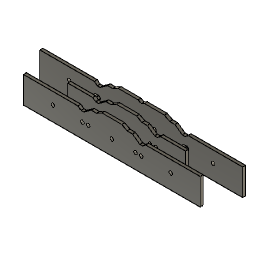
Spur_0_Module_Kopfstuecke_v3 (Autodesk Fusion 360 design; units mm, degrees)
Autodesk Fusion 360 part; units mm, degrees
sketch "Skizze1" plane through (0, 0, 0) normal (0, 1, 0) x (1, 0, 0) in component "FREMO_600mm"
  line L0 (0, 0) -> (0, -110) construction
  line L1 (0, 0) -> (-300, 0)
  line L2 (-300, 0) -> (-300, -90)
  line L3 (-300, -90) -> (-115, -90)
  line L4 (0, -110) -> (-34, -110)
  line L5 (-34, -110) -> (-52, -100)
  line L6 (-52, -100) -> (-70, -100)
  line L7 (-70, -100) -> (-95, -82)
  line L8 (-95, -82) -> (-105, -82)
  line L9 (-105, -82) -> (-115, -90)
  line L10 (-300, -50) -> (0, -50) construction
  circle A0 centre (-100, -50) radius 6
  circle A1 centre (-80, -50) radius 6
  circle A2 centre (-200, -50) radius 6
  line L11 (0, -110) -> (34, -110)
  line L12 (34, -110) -> (52, -100)
  line L13 (52, -100) -> (70, -100)
  line L14 (70, -100) -> (95, -82)
  line L15 (95, -82) -> (105, -82)
  line L16 (105, -82) -> (115, -90)
  line L17 (300, -90) -> (115, -90)
  line L18 (300, 0) -> (300, -90)
  line L19 (0, 0) -> (300, 0)
  circle A3 centre (200, -50) radius 6
  circle A4 centre (100, -50) radius 6
  circle A5 centre (80, -50) radius 6
  circle A6 centre (0, -50) radius 6
  dimension "d13" = 34
  dimension "d14" = 18
  dimension "d15" = 18
  dimension "d16" = 10
  dimension "d17" = 25
  dimension "d18" = 10
  dimension "d19" = 10
  dimension "d20" = 100
  dimension "d21" = 90
  dimension "d22" = 8
  dimension "d23" = 300
  dimension "d24" = 12
  dimension "d25" = 12
  dimension "d26" = 12
  dimension "d27" = 50
  dimension "d28" = 80
  dimension "d29" = 100
  dimension "d30" = 200
  dimension "d31" = 12
  constraint coincident L0.start L1.start
  constraint vertical L0
  constraint perpendicular L0 L1
  constraint perpendicular L1 L2
  constraint perpendicular L0 L4
  constraint parallel L4 L6
  constraint parallel L6 L8
  constraint parallel L3 L8
  constraint coincident L2 L10.start
  constraint coincident L0 L10.end
  constraint perpendicular L0 L10
  constraint coincident L10 A0.centre
  constraint coincident L10 A1.centre
  constraint coincident L10 A2.centre
  constraint symmetric L4.start L0 L11.start
  constraint symmetric L0 L1.start L19.start
  constraint symmetric L0 L1.end L18.start
  constraint symmetric L0 L2.end L17.start
  constraint symmetric L0 L3.end L16.end
  constraint symmetric L0 L4.end L11.end
  constraint symmetric L0 L5.end L12.end
  constraint symmetric L0 L6.end L13.end
  constraint symmetric L0 L7.end L14.end
  constraint symmetric L0 L8.end L15.end
  constraint symmetric L0 A0 A4
  constraint symmetric L0 A1 A5
  constraint symmetric L0 A2 A3
  constraint coincident L10.end A6.centre
  measures "d13" distance of L0.end L4.end
  measures "d14" horizontal distance of L4.end L5.end
  measures "d15" distance of L5.end L6.end
  measures "d16" distance of L4 L6
  measures "d17" horizontal distance of L6.end L7.end
  measures "d18" distance of L7.end L8.end
  measures "d19" horizontal distance of L3.end L8.end
  measures "d20" distance of L1 L6
  measures "d21" distance of L1 L3
  measures "d22" distance of L3 L8
  measures "d23" distance of L0 L2
  measures "d24" diameter of A0
  measures "d25" diameter of A1
  measures "d26" diameter of A2
  measures "d27" distance of L1 L10
  measures "d28" distance of L0 A1.centre
  measures "d29" distance of L0 A0.centre
  measures "d30" distance of L0 A2.centre
  measures "d31" diameter of A6
extrude "Extrusion1" add sketch "Skizze1" along normal blind 10 makes body 1 in component "FREMO_600mm"
sketch "Skizze2" plane through (0, 0, 0) normal (0, 1, 0) x (1, 0, 0) in component "FREMO_400mm"
  line L0 (0, 0) -> (0, -110) construction
  line L1 (0, 0) -> (-200, 0)
  line L2 (-200, 0) -> (-200, -90)
  line L3 (-200, -90) -> (-115, -90)
  line L4 (-115, -90) -> (-105, -82)
  line L5 (-105, -82) -> (-95, -82)
  line L6 (-95, -82) -> (-70, -100)
  line L7 (-70, -100) -> (-52, -100)
  line L8 (-52, -100) -> (-34, -110)
  line L9 (-34, -110) -> (0, -110)
  line L10 (-200, -50) -> (0, -50) construction
  circle A0 centre (-100, -50) radius 6
  circle A1 centre (-80, -50) radius 6
  line L11 (34, -110) -> (0, -110)
  line L12 (52, -100) -> (34, -110)
  line L13 (70, -100) -> (52, -100)
  line L14 (95, -82) -> (70, -100)
  line L15 (105, -82) -> (95, -82)
  line L16 (115, -90) -> (105, -82)
  line L17 (200, -90) -> (115, -90)
  line L18 (200, 0) -> (200, -90)
  line L19 (0, 0) -> (200, 0)
  circle A2 centre (100, -50) radius 6
  circle A3 centre (80, -50) radius 6
  circle A4 centre (0, -50) radius 6
  dimension "d52" = 34
  dimension "d53" = 18
  dimension "d54" = 18
  dimension "d55" = 25
  dimension "d56" = 10
  dimension "d57" = 10
  dimension "d58" = 10
  dimension "d59" = 100
  dimension "d60" = 90
  dimension "d61" = 8
  dimension "d62" = 200
  dimension "d63" = 50
  dimension "d64" = 12
  dimension "d65" = 12
  dimension "d66" = 80
  dimension "d67" = 100
  dimension "d68" = 12
  constraint coincident L0.start L1.start
  constraint vertical L0
  constraint perpendicular L0 L1
  constraint perpendicular L1 L2
  constraint perpendicular L0 L9
  constraint parallel L7 L9
  constraint parallel L5 L7
  constraint parallel L3 L5
  constraint coincident L2 L10.start
  constraint coincident L0 L10.end
  constraint perpendicular L0 L10
  constraint coincident L10 A0.centre
  constraint coincident L10 A1.centre
  constraint symmetric L9.end L0 L11.end
  constraint symmetric L0 L1.start L19.start
  constraint symmetric L0 L1.end L18.start
  constraint symmetric L0 L2.end L17.start
  constraint symmetric L0 L3.end L16.start
  constraint symmetric L0 L4.end L15.start
  constraint symmetric L0 L5.end L14.start
  constraint symmetric L0 L6.end L13.start
  constraint symmetric L0 L7.end L12.start
  constraint symmetric L0 L8.end L11.start
  constraint symmetric L0 A0 A2
  constraint symmetric L0 A1 A3
  constraint coincident L10.end A4.centre
  measures "d52" distance of L0.end L8.end
  measures "d53" horizontal distance of L7.end L8.end
  measures "d54" distance of L6.end L7.end
  measures "d55" horizontal distance of L5.end L6.end
  measures "d56" distance of L4.end L5.end
  measures "d57" horizontal distance of L3.end L4.end
  measures "d58" distance of L7 L9
  measures "d59" distance of L1 L7
  measures "d60" distance of L1 L3
  measures "d61" distance of L3 L5
  measures "d62" distance of L0 L2
  measures "d63" distance of L1 L10
  measures "d64" diameter of A0
  measures "d65" diameter of A1
  measures "d66" distance of L0 A1.centre
  measures "d67" distance of L0 A0.centre
  measures "d68" diameter of A4
extrude "Extrusion2" add sketch "Skizze2" along normal blind 10 separate body makes body 2 in component "FREMO_400mm"
sketch "Skizze1 (2)" plane through (0, 0, 0) normal (0, 1, 0) x (1, 0, 0) in component "FREMO_Entwurf_2_Gleisig_689mm"
  line L0 (0, 0) -> (0, -104.1667) construction
  line L1 (0, 0) -> (-344.5, 0)
  line L2 (-344.5, 0) -> (-344.5, -90)
  line L3 (-344.5, -90) -> (-159.5, -90)
  line L4 (-159.5, -90) -> (-149.5, -82)
  line L5 (-149.5, -82) -> (-139.5, -82)
  line L6 (-139.5, -82) -> (-114.5, -100)
  line L7 (-114.5, -100) -> (-96.5, -100)
  line L8 (-96.5, -100) -> (-78.5, -110)
  line L9 (-78.5, -110) -> (-10.5, -110)
  line L10 (-44.5, -110) -> (-44.5, 0) construction
  line L11 (-44.5, -50) -> (-344.5, -50) construction
  circle A0 centre (-44.5, -50) radius 6
  circle A1 centre (-144.5, -50) radius 6
  circle A2 centre (-244.5, -50) radius 6
  line L12 (-96.5, -100) -> (7.5, -100) construction
  line L13 (-10.5, -110) -> (0, -104.1667)
  line L14 (0, -104.1667) -> (7.5, -100) construction
  line L15 (10.5, -110) -> (0, -104.1667)
  line L16 (78.5, -110) -> (10.5, -110)
  line L17 (96.5, -100) -> (78.5, -110)
  line L18 (114.5, -100) -> (96.5, -100)
  line L19 (139.5, -82) -> (114.5, -100)
  line L20 (149.5, -82) -> (139.5, -82)
  line L21 (159.5, -90) -> (149.5, -82)
  line L22 (344.5, -90) -> (159.5, -90)
  line L23 (344.5, 0) -> (344.5, -90)
  line L24 (0, 0) -> (344.5, 0)
  line L25 (44.5, -50) -> (344.5, -50) construction
  circle A3 centre (244.5, -50) radius 6
  circle A4 centre (144.5, -50) radius 6
  circle A5 centre (44.5, -50) radius 6
  line L26 (44.5, -110) -> (44.5, 0) construction
  circle A6 centre (-155.5, -50) radius 6
  circle A7 centre (155.5, -50) radius 6
  line L27 (-155.5, -56) -> (-144.5, -56)
  line L28 (-155.5, -44) -> (-144.5, -44)
  line L29 (144.5, -56) -> (155.5, -56)
  line L30 (144.5, -44) -> (155.5, -44)
  dimension "d71" = 68
  dimension "d72" = 18
  dimension "d73" = 18
  dimension "d74" = 25
  dimension "d75" = 10
  dimension "d76" = 10
  dimension "d77" = 8
  dimension "d78" = 10
  dimension "d79" = 100
  dimension "d80" = 90
  dimension "d81" = 44.5
  dimension "d82" = 300
  dimension "d83" = 12
  dimension "d84" = 12
  dimension "d85" = 12
  dimension "d86" = 100
  dimension "d87" = 200
  dimension "d88" = 50
  dimension "d90" = 18
  dimension "d91" = 12
  dimension "d92" = 12
  dimension "d93" = 200
  dimension "d94" = 200
  constraint coincident L0.start L1.start
  constraint vertical L0
  constraint perpendicular L0 L1
  constraint perpendicular L1 L2
  constraint perpendicular L0 L9
  constraint parallel L7 L9
  constraint parallel L5 L7
  constraint parallel L3 L5
  constraint midpoint L9 L10.start
  constraint coincident L1 L10.end
  constraint perpendicular L1 L10
  constraint coincident L10 L11.start
  constraint coincident L2 L11.end
  constraint perpendicular L10 L11
  constraint coincident L11.start A0.centre
  constraint coincident L11 A1.centre
  constraint coincident L11 A2.centre
  constraint parallel L7 L12
  constraint coincident L0 L13.end
  constraint parallel L13 L14
  constraint coincident L0.end L13.end
  constraint symmetric L0 L1.start L24.start
  constraint symmetric L0 L1.end L23.start
  constraint symmetric L0 L2.end L22.start
  constraint symmetric L0 L3.end L21.start
  constraint symmetric L0 L4.end L20.start
  constraint symmetric L0 L5.end L19.start
  constraint symmetric L0 L6.end L18.start
  constraint symmetric L0 L7.end L17.start
  constraint symmetric L0 L8.end L16.start
  constraint symmetric L0 L9.end L15.start
  constraint symmetric L0 L10.start L26.start
  constraint symmetric L0 L10.end L26.end
  constraint symmetric L0 L11.start L25.start
  constraint symmetric L0 L11.end L25.end
  constraint symmetric L0 A0 A5
  constraint symmetric L0 A1 A4
  constraint symmetric L0 A2 A3
  constraint symmetric L0 L13.end L14.start
  constraint coincident L11 A6.centre
  constraint coincident L25 A7.centre
  constraint coincident A6 L27.start
  constraint coincident A1 L27.end
  constraint coincident A6 L28.start
  constraint coincident A1 L28.end
  constraint tangent A6 L27
  constraint tangent A1 L27
  constraint tangent A6 L28
  constraint tangent A1 L28
  constraint coincident A4 L29.start
  constraint coincident A7 L29.end
  constraint coincident A4 L30.start
  constraint coincident A7 L30.end
  constraint tangent A4 L29
  constraint tangent A7 L29
  constraint tangent A4 L30
  constraint tangent A7 L30
  measures "d71" distance of L8.end L9.end
  measures "d72" horizontal distance of L7.end L8.end
  measures "d73" distance of L6.end L7.end
  measures "d74" horizontal distance of L5.end L6.end
  measures "d75" distance of L4.end L5.end
  measures "d76" horizontal distance of L3.end L4.end
  measures "d77" distance of L3 L5
  measures "d78" distance of L7 L9
  measures "d79" distance of L1 L7
  measures "d80" distance of L1 L3
  measures "d81" distance of L0 L10
  measures "d82" distance of L2 L10
  measures "d83" diameter of A0
  measures "d84" diameter of A1
  measures "d85" diameter of A2
  measures "d86" distance of L10 A1.centre
  measures "d87" distance of L10 A2.centre
  measures "d88" distance of L1 L11
  measures "d90" horizontal distance of L9.end L12.end
  measures "d91" diameter of A6
  measures "d92" diameter of A7
  measures "d93" distance of L10 A7.centre
  measures "d94" distance of L26 A6.centre
extrude "Extrusion1'" add sketch "Skizze1 (2)" along normal blind 10 separate body makes body 3 in component "FREMO_Entwurf_2_Gleisig_689mm"
component "FREMO_600mm" placed x (1, 0, 0) y (0, 1, 0) z (0, 0, 1) at (0, 0, 0)
component "FREMO_400mm" placed x (1, 0, 0) y (0, 1, 0) z (0, 0, 1) at (0, 50, 0)
component "FREMO_Entwurf_2_Gleisig_689mm" placed x (1, 0, 0) y (0, 1, 0) z (0, 0, 1) at (0, 100, 0)
equation "d81 = ( 89 / 2 ) * 1 mm"
